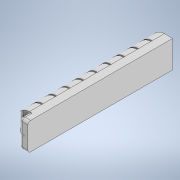
# Autodesk Inventor part: 3D_print_actuator
Saved by Autodesk Inventor 2021 (Build 250183000, 183)
## iProperties
Created: 2021-04-12
Part Number: 3D_print_actuator
Material: Generic
Document SubType Name: Modeling
Designer: Charlie
Density: 1 g/cm^3
Appearance: Default
Author: Charlie
Autodesk Inventor part; units mm, degrees
ref_plane "YZ Plane" through (0, 0, 0) normal (1, 0, 0) x (0, 1, 0)
ref_plane "XY Plane" through (0, 0, 0) normal (0, 0, 1) x (1, 0, 0)
sketch "Sketch1" plane through (0, 0, 0) normal (0, 1, 0) x (-1, 0, 0)
  line L0 (0, 0) -> (0, 100)
  line L1 (0, 0) -> (10.5, 0) construction
  line L2 (15, 4.5) -> (15, 4.5) construction
  line L3 (0, 0) -> (6, 0) construction
  line L4 (10.5, 9) -> (6, 9) construction
  line L5 (6, 9) -> (6, 10)
  line L6 (6, 0) -> (10.5, 0)
  line L7 (15, 9) -> (10.5, 9) construction
  line L8 (15, 9) -> (15, 0) construction
  arc A0 (10.5, 0) -> (15, 4.5) centre (10.5, 4.5) ccw
  arc A1 (15, 4.5) -> (10.5, 9) centre (10.5, 4.5) ccw
  line L9 (10.5, 0) -> (15, 0) construction
  line L10 (10.5, 9) -> (6, 9)
  line L11 (6, 19) -> (6, 20)
  arc A2 (10.5, 10) -> (15, 14.5) centre (10.5, 14.5) ccw
  arc A3 (15, 14.5) -> (10.5, 19) centre (10.5, 14.5) ccw
  line L12 (0, 10) -> (10.5, 10) construction
  line L13 (10.5, 19) -> (6, 19) construction
  line L14 (10.5, 19) -> (6, 19)
  line L15 (6, 10) -> (10.5, 10)
  line L16 (6, 29) -> (6, 30)
  arc A4 (10.5, 20) -> (15, 24.5) centre (10.5, 24.5) ccw
  arc A5 (15, 24.5) -> (10.5, 29) centre (10.5, 24.5) ccw
  line L17 (0, 20) -> (10.5, 20) construction
  line L18 (10.5, 29) -> (6, 29) construction
  line L19 (10.5, 29) -> (6, 29)
  line L20 (6, 20) -> (10.5, 20)
  line L21 (6, 39) -> (6, 40)
  arc A6 (10.5, 30) -> (15, 34.5) centre (10.5, 34.5) ccw
  arc A7 (15, 34.5) -> (10.5, 39) centre (10.5, 34.5) ccw
  line L22 (0, 30) -> (10.5, 30) construction
  line L23 (10.5, 39) -> (6, 39) construction
  line L24 (10.5, 39) -> (6, 39)
  line L25 (6, 30) -> (10.5, 30)
  line L26 (6, 49) -> (6, 50)
  arc A8 (10.5, 40) -> (15, 44.5) centre (10.5, 44.5) ccw
  arc A9 (15, 44.5) -> (10.5, 49) centre (10.5, 44.5) ccw
  line L27 (0, 40) -> (10.5, 40) construction
  line L28 (10.5, 49) -> (6, 49) construction
  line L29 (10.5, 49) -> (6, 49)
  line L30 (6, 40) -> (10.5, 40)
  line L31 (6, 59) -> (6, 60)
  arc A10 (10.5, 50) -> (15, 54.5) centre (10.5, 54.5) ccw
  arc A11 (15, 54.5) -> (10.5, 59) centre (10.5, 54.5) ccw
  line L32 (0, 50) -> (10.5, 50) construction
  line L33 (10.5, 59) -> (6, 59) construction
  line L34 (10.5, 59) -> (6, 59)
  line L35 (6, 50) -> (10.5, 50)
  line L36 (6, 69) -> (6, 70)
  arc A12 (10.5, 60) -> (15, 64.5) centre (10.5, 64.5) ccw
  arc A13 (15, 64.5) -> (10.5, 69) centre (10.5, 64.5) ccw
  line L37 (0, 60) -> (10.5, 60) construction
  line L38 (10.5, 69) -> (6, 69) construction
  line L39 (10.5, 69) -> (6, 69)
  line L40 (6, 60) -> (10.5, 60)
  line L41 (6, 79) -> (6, 80)
  arc A14 (10.5, 70) -> (15, 74.5) centre (10.5, 74.5) ccw
  arc A15 (15, 74.5) -> (10.5, 79) centre (10.5, 74.5) ccw
  line L42 (0, 70) -> (10.5, 70) construction
  line L43 (10.5, 79) -> (6, 79) construction
  line L44 (10.5, 79) -> (6, 79)
  line L45 (6, 70) -> (10.5, 70)
  line L46 (6, 89) -> (6, 90)
  arc A16 (10.5, 80) -> (15, 84.5) centre (10.5, 84.5) ccw
  arc A17 (15, 84.5) -> (10.5, 89) centre (10.5, 84.5) ccw
  line L47 (0, 80) -> (10.5, 80) construction
  line L48 (10.5, 89) -> (6, 89) construction
  line L49 (10.5, 89) -> (6, 89)
  line L50 (6, 80) -> (10.5, 80)
  line L51 (6, 99) -> (6, 100)
  arc A18 (10.5, 90) -> (15, 94.5) centre (10.5, 94.5) ccw
  arc A19 (15, 94.5) -> (10.5, 99) centre (10.5, 94.5) ccw
  line L52 (0, 90) -> (10.5, 90) construction
  line L53 (10.5, 99) -> (6, 99) construction
  line L54 (10.5, 99) -> (6, 99)
  line L55 (6, 90) -> (10.5, 90)
  line L56 (0, 100) -> (0, 106)
  line L57 (0, 106) -> (3, 106)
  line L58 (6, 103) -> (6, 100)
  line L59 (6, 0) -> (0, 0)
  line L60 (6, 103) -> (6, 106)
  line L61 (6, 106) -> (3, 106)
  point P0 (15, 10)
  point P1 (15, 19)
  point P2 (15, 20)
  point P3 (15, 29)
  point P4 (15, 30)
  point P5 (15, 39)
  point P6 (15, 40)
  point P7 (15, 49)
  point P8 (15, 50)
  point P9 (15, 59)
  point P10 (15, 60)
  point P11 (15, 69)
  point P12 (15, 70)
  point P13 (15, 79)
  point P14 (15, 80)
  point P15 (15, 89)
  point P16 (15, 90)
  point P17 (15, 99)
  dimension "d0" = 100
  dimension "d1" = 15
  dimension "d2" = 9
  dimension "d3" = 6
  dimension "d4" = 1
  dimension "d5" = 4.5
  dimension "d6" = 4.5
  dimension "d11" = 10
  dimension "d16" = 6
  dimension "d17" = 6
  constraints: 124 end point, 40 point on circle, 34 point on line, 20 centre point, 5 perpendicular, 5 vertical, 4 collinear, 4 tangent, 3 horizontal, 170 other
  measures "d0" distance of L0.start L0.end
  measures "d1" distance of L0.start L8.end
  measures "d2" distance of L8.end L7.start
  measures "d3" distance of L0.start L3.end
  measures "d4" distance of L4.end L5.end
  measures "d5" radius of A0
  measures "d6" radius of A1
  measures "d11" distance of L4.end L11.start
  measures "d16" distance of L0.end L56.end
  measures "d17" distance of L56.end L60.end
extrude "Extrusion1" add sketch "Sketch1" along normal blind 20
sketch "Sketch2" plane through (0, 0, 0) normal (0, 0, -1) x (-1, 0, 0)
  line L0 (15, 20) -> (10.5, 20) construction
  line L1 (6, 20) -> (0, 20)
  line L2 (0, 20) -> (0, 0)
  line L3 (0, 0) -> (6, 0)
  line L4 (15, 9) -> (15, 11)
  line L5 (15, 20) -> (0, 0) construction
  arc A0 (15, 11) -> (6, 20) centre (6, 11) ccw
  arc A1 (6, 0) -> (15, 9) centre (6, 9) ccw
  line L6 (-2, -4) -> (17, -4)
  line L7 (17, -4) -> (17, 24)
  line L8 (17, 24) -> (-2, 24)
  line L9 (-2, 24) -> (-2, -4)
  line L10 (-2, -4) -> (17, 24) construction
  line L11 (17, -4) -> (-2, 24) construction
  point P0 (15, 0)
  point P1 (7.5, 10)
  dimension "d21" = 15
  dimension "d22" = 20
  dimension "d23" = 9
  dimension "d24" = 9
  dimension "d25" = 19
  dimension "d26" = 28
  constraints: 22 end point, 4 parallel, 4 point on circle, 4 point on line, 4 tangent, 3 midpoint, 2 centre point, 2 horizontal, 2 perpendicular
  measures "d21" distance of L2.end point (15, 0)
  measures "d22" distance of L1.end L2.end
  measures "d23" radius of A0
  measures "d24" radius of A1
  measures "d25" distance of L8.end L7.end
  measures "d26" distance of L7.end L6.end
extrude "Extrusion2" cut sketch "Sketch2" against normal blind 100
shell "Shell2" thickness 1 removed faces 1 at (-4, 6.6667, 106)
sketch "Sketch7" plane through (-6, 0, 106) normal (0, 0, 1) x (1, 0, 0)
  line L0 (0, 20) -> (6, 20) projected
  line L1 (0, 0) -> (6, 0)
  line L2 (6, 0) -> (6, 20)
  line L3 (6, 20) -> (0, 20)
  line L4 (0, 20) -> (0, 0)
  circle A0 centre (3, 10) radius 0.5
  point P0 (6, 0)
  dimension "d46" = 1
  constraints: 8 end point, 2 parallel, 1 centre point, 1 horizontal, 1 perpendicular
  measures "d46" diameter of A0
extrude "Extrusion5" add sketch "Sketch7" against normal blind 8 contours L0 L2 L1 L4 | A0
fillet "Fillet2" radius 2 5 edges at (-6, 20, 102.5) (-6, 10, 106) (-6, 0, 102.5) (-3, 0, 106) (-3, 20, 106)
extrude "Extrusion6" cut sketch "Sketch7" against normal blind 2 contours A0
sketch "Sketch8" plane through (0, 0, 0) normal (1, 0, 0) x (0, 1, 0)
  line L0 (0, 9) -> (20, 9) projected
  line L1 (0, 10) -> (20, 10) projected
  line L2 (0, 9) -> (20, 9)
  line L3 (20, 9) -> (20, 10)
  line L4 (20, 10) -> (0, 10)
  line L5 (0, 10) -> (0, 9)
  line L6 (0, 19) -> (20, 19)
  line L7 (20, 20) -> (0, 20)
  line L8 (20, 19) -> (20, 20)
  line L9 (0, 20) -> (0, 19)
  line L10 (0, 29) -> (20, 29)
  line L11 (20, 30) -> (0, 30)
  line L12 (20, 29) -> (20, 30)
  line L13 (0, 30) -> (0, 29)
  line L14 (0, 39) -> (20, 39)
  line L15 (20, 40) -> (0, 40)
  line L16 (20, 39) -> (20, 40)
  line L17 (0, 40) -> (0, 39)
  line L18 (0, 49) -> (20, 49)
  line L19 (20, 50) -> (0, 50)
  line L20 (20, 49) -> (20, 50)
  line L21 (0, 50) -> (0, 49)
  line L22 (0, 59) -> (20, 59)
  line L23 (20, 60) -> (0, 60)
  line L24 (20, 59) -> (20, 60)
  line L25 (0, 60) -> (0, 59)
  line L26 (0, 69) -> (20, 69)
  line L27 (20, 70) -> (0, 70)
  line L28 (20, 69) -> (20, 70)
  line L29 (0, 70) -> (0, 69)
  line L30 (0, 79) -> (20, 79)
  line L31 (20, 80) -> (0, 80)
  line L32 (20, 79) -> (20, 80)
  line L33 (0, 80) -> (0, 79)
  line L34 (0, 89) -> (20, 89)
  line L35 (20, 90) -> (0, 90)
  line L36 (20, 89) -> (20, 90)
  line L37 (0, 90) -> (0, 89)
  point P0 (0, 0)
  dimension "d51" = 10
  constraints: 72 end point, 2 parallel, 1 collinear, 1 horizontal, 1 perpendicular, 1 vertical, 63 other
  measures "d51" distance of L0.start L6.start
extrude "Extrusion7" add sketch "Sketch8" against normal blind 6
ref_plane "Work Plane1" through (-6, 0, 99) normal (0, 0, 1) x (1, 0, 0)
sketch "Sketch4" plane through (-6, 0, 99) normal (0, 0, 1) x (1, 0, 0)
  line L0 (0, 0) -> (0, 20) projected
  line L1 (0, 0) -> (6, 20) construction
  circle A0 centre (3, 10) radius 2 construction
  line L2 (5, 6.5) -> (3, 6.5)
  line L3 (1, 8.5) -> (1, 11.5)
  line L4 (3, 13.5) -> (5, 13.5)
  line L5 (5, 13.5) -> (5, 6.5)
  line L6 (5, 6.5) -> (1, 13.5) construction
  line L7 (1, 6.5) -> (5, 13.5) construction
  arc A1 (3, 13.5) -> (1, 11.5) centre (3, 11.5) ccw
  arc A2 (1, 8.5) -> (3, 6.5) centre (3, 8.5) ccw
  point P0 (6, 0)
  point P1 (3, 10)
  point P2 (1, 10)
  point P3 (5, 10)
  dimension "d31" = 4
  dimension "d58" = 4
  dimension "d59" = 7
  dimension "d60" = 2
  constraints: 14 end point, 4 point on circle, 4 point on line, 4 tangent, 3 centre point, 3 midpoint, 2 parallel, 1 equal radius, 1 horizontal, 1 perpendicular
  measures "d31" diameter of A0
  measures "d58" distance of L6.end L4.end
  measures "d59" distance of L7.start L6.end
  measures "d60" radius of A1
extrude "Extrusion3" cut sketch "Sketch4" against normal blind 96
sketch "Sketch6" plane through (0, 10, 0) normal (0, 1, 0) x (-1, 0, 0)
  line L0 (21.0864, 109.726) -> (-9.863, 109.726)
  line L1 (-9.863, 109.726) -> (-9.863, -3.5286)
  line L2 (-9.863, -3.5286) -> (21.0864, -3.5286)
  line L3 (21.0864, -3.5286) -> (21.0864, 109.726)
  point P0 (0, 0)
  dimension "d36" = 113.2546
  dimension "d37" = 30.9494
  constraints: 8 end point, 2 parallel, 1 horizontal, 1 perpendicular
  measures "d36" distance of L2.end L0.start
  measures "d37" distance of L1.end L2.end
body "Solid1"
